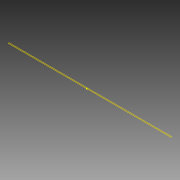
# Autodesk Inventor part: foam
Saved by Autodesk Inventor 2015 SP1 (Build 190203100, 203)
## iProperties
Created: 2015-02-12
Part Number: foam
Material: Generic
Document SubType Name: Modeling
Designer: Jostein
Density: 1 g/cm^3
Appearance: Default
Author: Jostein
Autodesk Inventor part; units mm, degrees
ref_plane "YZ Plane" through (0, 0, 0) normal (1, 0, 0) x (0, 1, 0)
ref_plane "XZ Plane" through (0, 0, 0) normal (0, 1, 0) x (-1, 0, 0)
ref_plane "XY Plane" through (0, 0, 0) normal (0, 0, 1) x (1, 0, 0)
sketch "Sketch3" plane through (0, 0, 0) normal (0, 0, 1) x (1, 0, 0)
  line L0 (254.9401, 3) -> (-235.0599, 3) construction
  line L1 (-235.0599, 0) -> (254.9401, 0) construction
  line L2 (254.9401, 0) -> (254.9401, 3) construction
  line L3 (-235.0599, 3) -> (-235.0599, 0)
  line L4 (-235.0599, 3) -> (-215.0599, 3)
  line L5 (-215.0599, 3) -> (-215.0599, 128)
  line L6 (-215.0599, 128) -> (-235.0599, 128)
  line L7 (-280.0599, 128) -> (-280.0599, 125)
  line L8 (-280.0599, 125) -> (-310.0599, 125)
  line L9 (-310.0599, 125) -> (-310.0599, 73)
  line L10 (9.9401, 200) -> (9.9401, 0) construction
  line L11 (-310.0599, 73) -> (-276.8239, 22.5087)
  arc A0 (-276.8239, 22.5087) -> (-235.0599, 0) centre (-235.0599, 50) ccw
  line L12 (-251.7655, 39.0035) -> (-280.0599, 81.9876)
  line L13 (-280.0599, 81.9876) -> (-280.0599, 125)
  arc A1 (-251.7655, 39.0035) -> (-248.9273, 35.5883) centre (-235.0599, 50) ccw
  line L14 (-215.0599, 3) -> (-248.9273, 35.5883)
  point P0 (0, 0)
  dimension "d0" = 20
  dimension "d1" = 125
  dimension "d2" = 65
  dimension "d3" = 3
  dimension "d4" = 30
  dimension "d5" = 70
  dimension "d9" = 490
  dimension "d10" = 200
  dimension "d11" = 245
  dimension "d15" = 50
  constraints: 26 end point, 4 perpendicular, 4 point on circle, 4 tangent, 3 vertical, 2 centre point, 2 point on line, 1 horizontal, 1 midpoint, 3 other
  measures "d0" distance of L0.end L4.end
  measures "d1" distance of L4.end L5.end
  measures "d2" distance of L5.end L7.start
  measures "d3" distance of L7.start L7.end
  measures "d4" distance of L7.end L8.end
  measures "d5" vertical distance of L0.end L9.end
  measures "d9" distance of L1.start L1.end
  measures "d10" distance of L10.start L10.end
  measures "d11" distance from line of L0.start L10
  measures "d15" radius of A0
revolve "Revolution1" add sketch "Sketch3" angle 360 about axis through (9.9401, 200, 0) along (0, -1, 0)
equation "\"d11\" = 0.5 * d9"
body "Solid1"
